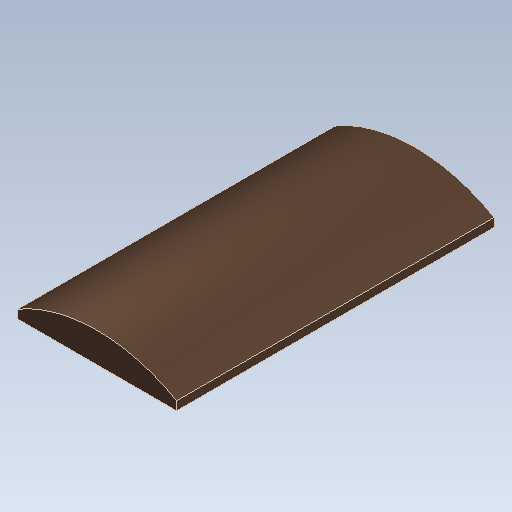
# Autodesk Inventor part: Башмак_CPY
Saved by Autodesk Inventor 2021 (Build 250183000, 183)
## iProperties
Created: 2020-11-29
Part Number: Башмак_CPY
Material: Бронза, мягкое олово
Document SubType Name: Modeling
Designer: Тимоха
Mass: 13316 g
Surface Area: 2491.73 cm^2
Volume: 1500.56 cm^3
Density: 8.874 g/cm^3
Appearance: Бронза - сатинированная
Author: Тимоха
Autodesk Inventor part; units mm, degrees
ref_plane "YZ Plane" through (0, 0, 0) normal (1, 0, 0) x (0, 1, 0)
sketch "Эскиз1" plane through (0, 0, 0) normal (0, 0, 1) x (1, 0, 0)
  circle A0 centre (0, 0) radius 175
  line L0 (0, 136) -> (87.5, 136)
  line L1 (87.5, 136) -> (-87.5, 136)
  line L2 (-87.5, 151.5544) -> (-87.5, 142)
  line L3 (-87.5, 142) -> (87.5, 142)
  line L4 (87.5, 142) -> (87.5, 151.5544)
  dimension "d0" = 350
  dimension "d1" = 87.5
  dimension "d2" = 175
  dimension "d13" = 142
  constraints: 10 end point, 2 perpendicular, 2 point on circle, 1 centre point, 1 coincident, 1 horizontal, 1 point on line, 1 vertical
  measures "d0" diameter of A0
  measures "d1" distance of L0.start L0.end
  measures "d2" distance of L0.end L1.end
  measures "d13" distance from line of point (0, 0) L3
extrude "Выдавливание1" add sketch "Эскиз1" along normal blind 350 contours L4 L3 L2 A0 picked at (0, 153)
ref_plane "РабПлоскость1" through (0, 0, 175) normal (0, 0, -1) x (-1, 0, 0)
sketch "Эскиз2" plane through (0, 0, 175) normal (0, 0, -1) x (-1, 0, 0)
  arc A0 (87.5, 151.5544) -> (-87.5, 151.5544) centre (0, 0) ccw projected
  line L0 (-87.5, 142) -> (-87.5, 151.5544) projected
  arc A1 (87.5, 151.5544) -> (-87.5, 151.5544) centre (0, 0) ccw projected
  line L1 (87.5, 151.5544) -> (87.5, 142) projected
  line L2 (87.5, 142) -> (-87.5, 142) projected
  circle A2 centre (0, 0) radius 162.5
  line L3 (87.5, 142) -> (-87.5, 142) projected
  line L4 (0, 142) -> (-6, 142)
  line L5 (-6, 142) -> (-6, 162.3892)
  line L6 (0, 142) -> (6, 142)
  line L7 (6, 142) -> (6, 162.3892)
  point P0 (-79.0079, 142)
  point P1 (79.0079, 142)
  dimension "d7" = 325
  dimension "d8" = 6
  dimension "d9" = 6
  constraints: 8 end point, 2 point on circle, 2 point on line, 1 centre point, 1 coincident, 1 midpoint, 1 perpendicular
  measures "d7" diameter of A2
  measures "d8" distance of L4.start L4.end
  measures "d9" distance of L4.start L6.end
extrude "Выдавливание2" cut sketch "Эскиз2" against normal mid plane 320 contours L2 L7 A2 | A2 L5 L2
fillet "Сопряжение1" radius 5 10 edges at (-43.7095, 156.5111, 335) (43.7095, 156.5111, 335) (-6, 162.3892, 175) (-6, 152.1946, 335) (6, 162.3892, 175) (6, 152.1946, 335) (6, 152.1946, 15) (43.7095, 156.5111, 15) (-43.7095, 156.5111, 15) (-6, 152.1946, 15)
sketch "Эскиз3" plane through (-87.5, 142, 0) normal (0, -1, 0) x (1, 0, 0)
  line L0 (175, 0) -> (175, 8)
  line L1 (175, 0) -> (175, 350) projected
  line L2 (175, 8) -> (167, 8)
  dimension "d14" = 8
  constraints: 4 end point, 1 horizontal, 1 point on line
  measures "d14" distance of L0.start L0.end
hole "Отверстие1" at (79.5, 142, 8) direction (0, 1, 0) diameter 5 depth 8 tip angle 118 counterbore diameter 6 counterbore depth 6
mirror "Зеркальное отражение1" about plane through (0, 0, 0) normal (1, 0, 0) of "Отверстие1"
ref_plane "РабПлоскость2" through (0, 0, 175) normal (0, 0, -1) x (-1, 0, 0)
mirror "Зеркальное отражение2" about plane through (0, 0, 175) normal (0, 0, -1) of "Отверстие1", "Зеркальное отражение1"
thread "Резьба1" size "M6x1" class "6H" standard "ANSI Metric M Profile" full length
thread "Резьба2" size "M6x1" class "6H" standard "ANSI Metric M Profile" full length
thread "Резьба3" size "M6x1" class "6H" standard "ANSI Metric M Profile" full length
thread "Резьба4" size "M6x1" class "6H" standard "ANSI Metric M Profile" full length
